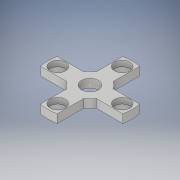
# Autodesk Inventor part: Disk-3
Saved by Autodesk Inventor 2019 (Build 230136000, 136)
## iProperties
Created: 2020-02-07
Part Number: Disk-3
Material: Generic
Document SubType Name: Modeling
Designer: gfb14170
Density: 1 g/cm^3
Appearance: Default
Author: gfb14170
Autodesk Inventor part; units mm, degrees
ref_plane "YZ Plane" through (0, 0, 0) normal (1, 0, 0) x (0, 1, 0)
ref_plane "XZ Plane" through (0, 0, 0) normal (0, 1, 0) x (-1, 0, 0)
ref_plane "XY Plane" through (0, 0, 0) normal (0, 0, 1) x (1, 0, 0)
sketch "Sketch1" plane through (0, 0, 0) normal (0, 1, 0) x (-1, 0, 0)
  circle A0 centre (0, 0) radius 3
  circle A1 centre (0, 0) radius 6 construction
  circle A2 centre (0, 0) radius 15 construction
  line L0 (-3, 14.6969) -> (-3, 5.1962)
  line L1 (3, 5.2197) -> (3, 14.6969)
  arc A3 (3, 14.6969) -> (-3, 14.6969) centre (0, 0) ccw
  line L2 (-5.2197, 3) -> (-14.6969, 3)
  arc A4 (-14.6969, 3) -> (-14.6969, -3) centre (0, 0) ccw
  line L3 (-14.6969, -3) -> (-5.1962, -3)
  line L4 (-3, -5.2197) -> (-3, -14.6969)
  arc A5 (-3, -14.6969) -> (3, -14.6969) centre (0, 0) ccw
  line L5 (3, -14.6969) -> (3, -5.1962)
  line L6 (5.2197, -3) -> (14.6969, -3)
  arc A6 (14.6969, -3) -> (14.6969, 3) centre (0, 0) ccw
  line L7 (14.6969, 3) -> (5.1962, 3)
  arc A7 (5.1962, 3) -> (3, 5.2197) centre (-0.2008, -0.1435) ccw
  arc A8 (3, -5.1962) -> (5.2197, -3) centre (-0.1229, 0.18) ccw
  arc A9 (-3, 5.1962) -> (-5.2197, 3) centre (0.1893, -0.2471) ccw
  arc A10 (-5.1962, -3) -> (-3, -5.2197) centre (0.2474, 0.1896) ccw
  dimension "d1" = 12
  dimension "d0" = 6
  dimension "d2" = 30
  dimension "d3" = 3
  dimension "d4" = 3
  dimension "d5" = 14.6969
  dimension "d8" = 360
  constraints: 18 point on circle, 16 end point, 10 centre point, 5 coincident, 1 concentric, 1 parallel, 34 other
  measures "d0" diameter of A0
  measures "d2" diameter of A2
  measures "d3" distance from line of point (0, 0) L1
  measures "d4" distance from line of point (0, 0) L0
  measures "d5" vertical distance of A2.centre L1.end
extrude "Extrusion1" add sketch "Sketch1" along normal blind 3
sketch "Sketch2" plane through (0, 3, 0) normal (0, 1, 0) x (1, 0, 0)
  circle A0 centre (0, -11.5) radius 2.75
  circle A1 centre (11.5, 0) radius 2.75
  circle A2 centre (0, 11.5) radius 2.75
  circle A3 centre (-11.5, 0) radius 2.75
  point P0 (0, 0)
  point P1 (11.5, 0)
  point P2 (0, 11.5)
  point P3 (-11.5, 0)
  dimension "d12" = 5.5
  dimension "d13" = 11.5
  dimension "d16" = 360
  dimension "d18" = 0
  dimension "d24" = 360
  constraints: 4 centre point, 14 other
  measures "d12" diameter of A0
  measures "d13" distance of point (0, 0) A0.centre
  measures "d18" horizontal distance of point (0, 0) A0.centre
sketch "Sketch3" plane through (0, 3, 0) normal (0, 1, 0) x (1, 0, 0)
  point P0 (0, 0)
extrude "Extrusion2" cut sketch "Sketch2" against normal blind 2
equation "\"d4\" = d3"
body "Solid1"
